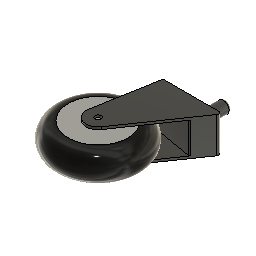
Roue_Folle (Autodesk Fusion 360 design; units mm, degrees)
Autodesk Fusion 360 part; units mm, degrees
sketch "Sketch1" plane through (0, 0, 0) normal (0, 0, 1) x (1, 0, 0)
  circle A0 centre (0, 0) radius 37.5
  dimension "d1" = 75
  constraint coincident A0.centre origin
  measures "d1" diameter of A0
extrude "Extrude1" add sketch "Sketch1" along normal blind 25 makes body 1
fillet "Fillet1" radius 12.5 2 edges at (-34.9623, -13.5606, 25) (-34.9623, -13.5606, 0) on bodies 1
copy_body "Body->Comp1" bodies 1 removing the originals makes body 2 in component "Component"
sketch "Sketch2" plane through (0, 0, 0) normal (0, 0, 1) x (1, 0, 0)
  circle A0 centre (0, 0) radius 10
  line L0 (-9.8481, 1.7365) -> (-0.4563, 55)
  line L1 (-0.4563, 55) -> (50, 55)
  line L2 (50, 55) -> (8.2371, -5.6701)
  circle A1 centre (0, 0) radius 2.5
  dimension "d6" = 20
  dimension "d7" = 55
  dimension "d8" = 50
  dimension "d9" = 100
  dimension "d14" = 5
  constraint coincident A0.centre A1.centre
  constraint coincident A0 L0.start
  constraint horizontal L1
  constraint coincident A0 L2.end
  constraint tangent A0 L2
  constraint tangent A0 L0
  constraint concentric A0 A1
  measures "d6" diameter of A0
  measures "d7" distance of A0.centre L1
  measures "d8" horizontal distance of A0.centre L1.end
  measures "d9" angle of L0 L1
  measures "d14" diameter of A1
extrude "Extrude2" add sketch "Sketch2" along normal blind 30 separate body makes body 3
sketch "Sketch3" plane through (-9.8481, 1.7365, 0) normal (-0.984808, 0.173648, 0) x (-0.173648, -0.984808, 0)
  line L0 (-54.0852, 0) -> (0, 0)
  line L1 (0, 0) -> (0, 30)
  line L2 (0, 30) -> (-54.0852, 30)
  line L3 (-54.0852, 30) -> (-54.0852, 0)
  line L4 (44.0852, 2) -> (-44.0852, 2)
  line L5 (-44.0852, 2) -> (-44.0852, 28)
  line L6 (-44.0852, 28) -> (44.0852, 28)
  line L7 (44.0852, 28) -> (44.0852, 2)
  line L8 (44.0852, 2) -> (-44.0852, 28) construction
  line L9 (-44.0852, 2) -> (44.0852, 28) construction
  point P0 (0, 15)
  dimension "d12" = 2
  dimension "d13" = 10
  constraint horizontal L4
  constraint perpendicular L4 L5
  constraint parallel L4 L6
  constraint parallel L5 L7
  constraint coincident L8 P0
  constraint coincident L9 P0
  constraint midpoint L1 P0
  measures "d12" distance of L2 L6
  measures "d13" horizontal distance of L0.start L4.end
extrude "Extrude3" cut sketch "Sketch3" against normal through all contours L1 L4 L5 L6 | L1 L4 L6 L7 bodies 3
sketch "Sketch4" plane through (0, 55, 0) normal (0, 1, 0) x (-1, 0, 0)
  line L0 (-50, 0) -> (0.4563, 0)
  line L1 (0.4563, 0) -> (0.4563, 30)
  line L2 (0.4563, 30) -> (-50, 30)
  line L3 (-50, 30) -> (-50, 0)
  line L4 (0.4563, 15) -> (-50, 15) construction
  circle A0 centre (-30, 15) radius 5
  dimension "d16" = 10
  dimension "d17" = 30
  constraint midpoint L1 L4.start
  constraint midpoint L3 L4.end
  constraint coincident L4 A0.centre
  measures "d16" diameter of A0
  measures "d17" horizontal distance of origin A0.centre
extrude "Extrude4" add sketch "Sketch4" along normal blind 22 contours A0 bodies 3
fillet "Fillet2" radius 2 1 edges at (50, 55, 15) on bodies 3
fillet "Fillet3" radius 2 1 edges at (34.6616, 77, 13.1919) on bodies 3
fillet "Fillet4" radius 1 2 edges at (38.3054, 38.011, 15) (-2.1928, 45.1519, 15) on bodies 3
copy_body "Body->Comp2" bodies 3 removing the originals makes body 4 in component "Component'"
component "Component" placed x (1, 0, 0) y (0, 1, 0) z (0, 0, 1) at (0, 0, 2.5)
component "Component'" placed x (1, 0, 0) y (0, 1, 0) z (0, 0, 1) at (0, 0, 0)
